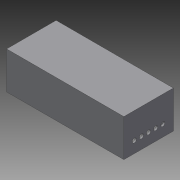
# Autodesk Inventor part: Case Botom v2
Saved by Autodesk Inventor 2015 (Build 190159000, 159)
## iProperties
Created: 2017-11-24
Part Number: Case Botom v2
Material: Generic
Document SubType Name: Modeling
Designer: Toby
Density: 1 g/cm^3
Appearance: Default
Author: Toby
Autodesk Inventor part; units mm, degrees
ref_plane "YZ Plane" through (0, 0, 0) normal (1, 0, 0) x (0, 1, 0)
ref_plane "XZ Plane" through (0, 0, 0) normal (0, 1, 0) x (-1, 0, 0)
ref_plane "XY Plane" through (0, 0, 0) normal (0, 0, 1) x (1, 0, 0)
sketch "Sketch1" plane through (0, 0, 0) normal (0, 0, 1) x (1, 0, 0)
  line L0 (-78.24, 3.5741) -> (4.16, 3.5741)
  line L1 (4.16, 3.5741) -> (4.16, -28.8259)
  line L2 (4.16, -28.8259) -> (-78.24, -28.8259)
  line L3 (-78.24, -28.8259) -> (-78.24, 3.5741)
  line L4 (-77.04, 2.3741) -> (2.96, 2.3741)
  line L5 (2.96, 2.3741) -> (2.96, -27.6259)
  line L6 (2.96, -27.6259) -> (-77.04, -27.6259)
  line L7 (-77.04, -27.6259) -> (-77.04, 2.3741)
  point P0 (0, 0)
  dimension "d0" = 32.4
  dimension "d1" = 82.4
  dimension "d2" = 1.2
  dimension "d3" = 1.2
  dimension "d4" = 1.2
  dimension "d5" = 1.2
  constraints: 16 end point, 4 parallel, 2 horizontal, 2 perpendicular
  measures "d0" distance of L0.end L1.end
  measures "d1" distance of L0.start L0.end
  measures "d2" distance between parallel lines of L4 L0
  measures "d3" distance between parallel lines of L2 L6
  measures "d4" distance between parallel lines of L7 L3
  measures "d5" distance between parallel lines of L1 L5
extrude "Extrusion1" add sketch "Sketch1" along normal blind 25
sketch "Sketch2" plane through (0, 0, 25) normal (0, 0, 1) x (1, 0, 0)
  line L0 (-78.24, 3.5741) -> (4.16, 3.5741)
  line L1 (4.16, 3.5741) -> (4.16, -28.8259)
  line L2 (4.16, -28.8259) -> (-78.24, -28.8259)
  line L3 (-78.24, -28.8259) -> (-78.24, 3.5741)
  point P0 (0, 0)
  constraints: 8 end point, 2 parallel, 1 horizontal, 1 perpendicular
extrude "Extrusion2" add sketch "Sketch2" along normal blind 1.2
sketch "Sketch3" plane through (-78.24, -28.8259, 0) normal (-1, 0, 0) x (0, 0, 1)
  line L0 (25, 1.2) -> (25, 31.2) projected
  line L1 (25, 12.45) -> (22, 12.45)
  line L2 (22, 12.45) -> (22, 19.95)
  line L3 (22, 19.95) -> (25, 19.95)
  line L4 (25, 19.95) -> (25, 12.45)
  line L5 (0, 1.2) -> (25, 1.2) projected
  line L6 (0, 31.2) -> (25, 31.2) projected
  point P0 (0, 28.8259)
  dimension "d10" = 7.5
  dimension "d11" = 3
  dimension "d12" = 11.25
  dimension "d13" = 11.25
  constraints: 8 end point, 2 parallel, 1 horizontal, 1 perpendicular, 1 point on line
  measures "d10" distance of L1.end L2.end
  measures "d11" distance of L2.end L3.end
  measures "d12" distance between parallel lines of L5 L1
  measures "d13" distance between parallel lines of L6 L3
extrude "Extrusion3" cut sketch "Sketch3" against normal blind 1.2
sketch "Sketch4" plane through (0, 0, 25) normal (0, 0, -1) x (-1, 0, 0)
  point P0 (0, 0)
sketch "Sketch5" plane through (0, 0, 25) normal (0, 0, -1) x (-1, 0, 0)
  line L0 (18.04, -7.6259) -> (19.04, -7.6259)
  line L1 (19.04, -7.6259) -> (19.04, -17.6259)
  line L2 (19.04, -17.6259) -> (18.04, -17.6259)
  line L3 (18.04, -17.6259) -> (18.04, -7.6259)
  line L4 (-2.96, 2.3741) -> (77.04, 2.3741) projected
  line L5 (77.04, -27.6259) -> (-2.96, -27.6259) projected
  line L6 (77.04, 2.3741) -> (77.04, -27.6259) projected
  point P0 (0, 0)
  dimension "d16" = 1
  dimension "d17" = 10
  dimension "d18" = 10
  dimension "d19" = 10
  dimension "d20" = 58
  constraints: 8 end point, 2 parallel, 1 horizontal, 1 perpendicular
  measures "d16" distance between parallel lines of L1 L3
  measures "d17" vertical distance of L2.end L0.end
  measures "d18" distance from line of L4 L0.start
  measures "d19" distance between parallel lines of L5 L2
  measures "d20" distance between parallel lines of L6 L1
extrude "Extrusion4" add sketch "Sketch5" along normal blind 1.5
chamfer "Chamfer1" distance 1.5 angle 45 2 edges at (-18.54, -17.6259, 23.5) (-18.54, -7.6259, 23.5)
chamfer "Chamfer2" distance 1.5 angle 45 1 edges at (-18.04, -12.6259, 25)
sketch "Sketch6" plane through (-78.24, -28.8259, 0) normal (0, -1, 0) x (1, 0, 0)
  circle A0 centre (3.7, 12.5) radius 2.5
  line L0 (1.2, 0) -> (1.2, 25) projected
  point P0 (78.24, 0)
  dimension "d29" = 5
  dimension "d30" = 2.5
  constraints: 1 centre point
  measures "d29" diameter of A0
  measures "d30" distance from line of L0 A0.centre
extrude "Extrusion5" cut sketch "Sketch6" against normal blind 40
sketch "Sketch7" plane through (4.16, -28.8259, 0) normal (1, 0, 0) x (0, 0, -1)
  line L0 (0, 31.2) -> (-25, 31.2) projected
  line L1 (0, 32.4) -> (0, 0) projected
  circle A0 centre (-8, 26.2) radius 1.5
  circle A1 centre (-8, 21.2) radius 1.5
  circle A2 centre (-8, 16.2) radius 1.5
  circle A3 centre (-8, 11.2) radius 1.5
  circle A4 centre (-8, 6.2) radius 1.5
  line L2 (0, 1.2) -> (-25, 1.2) projected
  point P0 (0, 28.8259)
  point P1 (-8, 31.2)
  dimension "d33" = 8
  dimension "d34" = 3
  dimension "d35" = 3
  dimension "d36" = 3
  dimension "d37" = 3
  dimension "d38" = 3
  dimension "d39" = 5
  dimension "d40" = 5
  dimension "d41" = 5
  dimension "d42" = 5
  dimension "d43" = 5
  dimension "d44" = 5
  constraints: 5 centre point, 1 point on line
  measures "d33" distance from line of L1 point (-8, 31.2)
  measures "d34" diameter of A0
  measures "d35" diameter of A1
  measures "d36" diameter of A2
  measures "d37" diameter of A3
  measures "d38" diameter of A4
  measures "d39" distance of A0.centre point (-8, 31.2)
  measures "d40" distance of A1.centre A0.centre
  measures "d41" distance of A2.centre A1.centre
  measures "d42" distance of A3.centre A2.centre
  measures "d43" distance of A4.centre A3.centre
  measures "d44" distance from line of L2 A4.centre
extrude "Extrusion6" cut sketch "Sketch7" against normal blind 3
sketch "Sketch8" plane through (0, 0, 0) normal (0, 0, -1) x (-1, 0, 0)
  line L0 (78.24, -28.8259) -> (-4.16, -28.8259)
  line L1 (-4.16, -28.8259) -> (-4.16, -30.0259)
  line L2 (-4.16, -30.0259) -> (78.24, -30.0259)
  line L3 (78.24, -30.0259) -> (78.24, -28.8259)
  line L4 (78.24, 3.5741) -> (-4.16, 3.5741)
  line L5 (-4.16, 3.5741) -> (-4.16, 4.7741)
  line L6 (-4.16, 4.7741) -> (78.24, 4.7741)
  line L7 (78.24, 4.7741) -> (78.24, 3.5741)
  line L8 (-4.16, 3.5741) -> (-4.16, -28.8259) projected
  point P0 (0, 0)
  dimension "d47" = 1.2
  dimension "d48" = 1.2
  constraints: 16 end point, 4 parallel, 2 collinear, 2 horizontal, 2 perpendicular
  measures "d47" distance of L1.end L0.end
  measures "d48" distance of L4.end L5.end
extrude "Extrusion7" add sketch "Sketch8" against normal blind 26.2
sketch "Sketch9" plane through (0, 0, 0) normal (0, 0, -1) x (-1, 0, 0)
  line L0 (-2.96, -27.6259) -> (77.04, -27.6259)
  line L1 (77.04, -27.6259) -> (77.04, -28.8259)
  line L2 (77.04, -28.8259) -> (-2.96, -28.8259)
  line L3 (-2.96, -28.8259) -> (-2.96, -27.6259)
  line L4 (77.04, 2.3741) -> (-2.96, 2.3741)
  line L5 (-2.96, 2.3741) -> (-2.96, 3.5741)
  line L6 (-2.96, 3.5741) -> (77.04, 3.5741)
  line L7 (77.04, 3.5741) -> (77.04, 2.3741)
  line L8 (-2.96, 2.3741) -> (77.04, 2.3741) projected
  line L9 (77.04, 2.3741) -> (77.04, -27.6259) projected
  point P0 (0, 0)
  dimension "d51" = 1.2
  dimension "d52" = 1.2
  constraints: 16 end point, 4 parallel, 2 collinear, 2 horizontal, 2 perpendicular, 2 point on line
  measures "d51" distance of L0.end L1.end
  measures "d52" distance of L4.end L5.end
extrude "Extrusion8" cut sketch "Sketch9" against normal blind 25
sketch "Sketch10" plane through (-78.24, -30.0259, 0) normal (-1, 0, 0) x (0, 0, 1)
  line L0 (25, 21.15) -> (25, 33.6) projected
  line L1 (22, 13.45) -> (25, 13.45)
  line L2 (25, 13.45) -> (25, 21.35)
  line L3 (25, 21.35) -> (22, 21.35)
  line L4 (22, 21.35) -> (22, 13.45)
  line L5 (25, 13.65) -> (22, 13.65) projected
  line L6 (22, 21.15) -> (25, 21.15) projected
  line L7 (22, 13.65) -> (22, 21.15) projected
  point P0 (0, 30.0259)
  dimension "d55" = 0.2
  dimension "d56" = 0.2
  constraints: 8 end point, 2 parallel, 1 collinear, 1 horizontal, 1 perpendicular, 1 point on line
  measures "d55" distance between parallel lines of L1 L5
  measures "d56" distance between parallel lines of L3 L6
extrude "Extrusion9" cut sketch "Sketch10" against normal blind 2
sketch "Sketch11" plane through (0, 0, 25) normal (0, 0, -1) x (-1, 0, 0)
  point P0 (0, 0)
body "Solid1"
